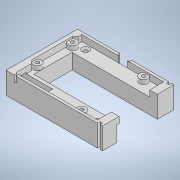
# Autodesk Inventor part: Стойка под электроннику
Saved by Autodesk Inventor 2020 (Build 240168000, 168)
## iProperties
Created: 2021-04-05
Part Number: Стойка под электроннику
Material: Типовые
Document SubType Name: Modeling
Designer: Антон
Density: 1 g/cm^3
Appearance: По умолчанию
Author: Антон
Autodesk Inventor part; units mm, degrees
ref_plane "YZ Plane" through (0, 0, 0) normal (1, 0, 0) x (0, 1, 0)
ref_plane "XZ Plane" through (0, 0, 0) normal (0, 1, 0) x (-1, 0, 0)
ref_plane "XY Plane" through (0, 0, 0) normal (0, 0, 1) x (1, 0, 0)
sketch "Эскиз1" plane through (0, 0, 0) normal (0, 1, 0) x (-1, 0, 0)
  line L0 (0, 0) -> (78, 0)
  line L1 (78, 0) -> (78, -57.8)
  line L2 (78, -57.8) -> (0, -57.8)
  line L3 (0, -57.8) -> (0, 0)
  line L4 (0, -28.9) -> (34.5, -28.9)
  line L5 (69, -13.4) -> (0, -13.4)
  line L6 (0, -13.4) -> (0, -44.4)
  line L7 (0, -44.4) -> (69, -44.4)
  line L8 (69, -44.4) -> (69, -13.4)
  line L9 (69, -13.4) -> (0, -44.4) construction
  line L10 (0, -13.4) -> (69, -44.4) construction
  line L11 (0, -13.4) -> (4, -13.4)
  point P0 (0, -13.4)
  dimension "d0" = 78
  dimension "d1" = 57.8
  dimension "d3" = 31
  dimension "d4" = 69
  constraints: 24 end point, 4 horizontal, 4 parallel, 3 midpoint, 2 perpendicular, 1 point on line
  measures "d0" distance of L1.end L2.end
  measures "d1" distance of L0.end L1.end
  measures "d3" distance of L6.end L5.end
  measures "d4" distance of L6.end L7.end
extrude "Выдавливание1" add sketch "Эскиз1" along normal blind 17.5 contours L0 L1 L2 L3 L7 L8 L5
sketch "Эскиз2" plane through (0, 17.5, 0) normal (0, 1, 0) x (1, 0, 0)
  line L0 (0, 0) -> (0, 2.05)
  line L1 (0, 0) -> (0, 57.8) projected
  line L2 (0, 2.05) -> (-6.2, 2.05)
  line L3 (-6.2, 2.05) -> (-72.4, 2.05)
  line L4 (-72.4, 2.05) -> (-72.4, 55.75)
  line L5 (-72.4, 55.75) -> (-6.2, 55.75)
  line L6 (-6.2, 55.75) -> (-6.2, 2.05)
  line L7 (-72.4, 2.05) -> (-72.4, 17.65)
  line L8 (-72.4, 17.65) -> (-74.9, 17.65)
  line L9 (-74.9, 17.65) -> (-74.9, 50.35)
  line L10 (-74.9, 50.35) -> (-72.4, 50.35)
  line L11 (-72.4, 50.35) -> (-72.4, 17.65)
  line L12 (-78, 57.8) -> (-78, 0) projected
  line L13 (-78, 0) -> (0, 0) projected
  point P0 (0, 11.4)
  point P1 (-72.4, 50.35)
  dimension "d9" = 2.05
  dimension "d10" = 6.2
  dimension "d11" = 66.2
  dimension "d12" = 53.7
  dimension "d13" = 15.6
  dimension "d14" = 2.5
  dimension "d15" = 32.7
  dimension "d16" = 57.8
  dimension "d17" = 78
  constraints: 22 end point, 4 parallel, 3 perpendicular, 2 horizontal, 2 point on line
  measures "d9" distance of L0.start L0.end
  measures "d10" distance of L0.end L2.end
  measures "d11" distance of L4.end L5.end
  measures "d12" distance of L3.end L4.end
  measures "d13" distance of L3.end L7.end
  measures "d14" distance of L9.end L10.end
  measures "d15" distance of L8.end L9.end
  measures "d16" distance of L12.start L12.end
  measures "d17" distance of L12.end L0.start
extrude "Выдавливание2" cut sketch "Эскиз2" against normal blind 5
sketch "Эскиз3" plane through (0, 12.5, 0) normal (0, 1, 0) x (1, 0, 0)
  line L0 (-74.9, 17.65) -> (-74.9, 50.35) projected
  line L1 (-74.9, 50.35) -> (-74.9, 48.15)
  line L2 (-74.9, 48.15) -> (-72.3, 48.15)
  circle A0 centre (-72.3, 48.15) radius 3.5
  line L3 (-74.9, 17.65) -> (-74.9, 19.65)
  line L4 (-74.9, 19.65) -> (-72.3, 19.65)
  circle A1 centre (-72.3, 19.65) radius 3.3
  line L5 (-6.2, 2.05) -> (-72.4, 2.05) projected
  line L6 (-6.2, 55.75) -> (-6.2, 2.05) projected
  line L7 (-6.2, 55.75) -> (-19.8, 55.75)
  line L8 (-72.4, 55.75) -> (-6.2, 55.75) projected
  line L9 (-19.8, 55.75) -> (-19.8, 53.15)
  circle A2 centre (-19.8, 53.15) radius 3.5
  line L10 (-6.2, 2.05) -> (-72.4, 2.05) projected
  line L11 (-6.2, 2.05) -> (-21.3, 2.05)
  line L12 (-21.3, 2.05) -> (-21.3, 4.65)
  circle A3 centre (-21.3, 4.65) radius 3.5
  point P0 (-6.2, 44.4)
  dimension "d26" = 2.2
  dimension "d27" = 2.6
  dimension "d28" = 7
  dimension "d29" = 2
  dimension "d30" = 2.6
  dimension "d31" = 6.6
  dimension "d35" = 13.6
  dimension "d36" = 2.6
  dimension "d37" = 7
  dimension "d38" = 15.1
  dimension "d39" = 2.6
  dimension "d40" = 7
  constraints: 16 end point, 4 centre point, 4 coincident, 4 point on line, 2 horizontal, 2 vertical
  measures "d26" distance of L0.end L1.end
  measures "d27" distance of L1.end L2.end
  measures "d28" diameter of A0
  measures "d29" distance of L0.start L3.end
  measures "d30" distance of L3.end L4.end
  measures "d31" diameter of A1
  measures "d35" distance of L6.start L7.end
  measures "d36" distance of L7.end L9.end
  measures "d37" diameter of A2
  measures "d38" distance of L5.start L11.end
  measures "d39" distance of L11.end L12.end
  measures "d40" diameter of A3
extrude "Выдавливание5" add sketch "Эскиз3" along normal blind 3.5
chamfer "Фаска2" distance 1 angle 45 1 edges at (-72.4, 15, -2.05)
chamfer "Фаска3" distance 2.5 angle 45 2 edges at (-72.4, 16.75, -17.65) (-72.4, 16.75, -50.35)
sketch "Эскиз4" plane through (-71.3, 16, -19.65) normal (0, 1, 0) x (0, 0, -1)
  arc A0 (-17.6, -52.3431) -> (-17.6, -47.6569) centre (-15, -50) ccw projected
  arc A1 (36.1, -49.1569) -> (36.1, -53.8431) centre (33.5, -51.5) ccw projected
  arc A2 (26.1569, 3.6) -> (31.5042, 2.7958) centre (28.5, 1) ccw projected
  arc A3 (-2.6937, 2.9063) -> (2.0322, 3.6) centre (0, 1) ccw projected
  point P0 (-19.65, -71.3)
  point P1 (50.1, -17.6)
  point P2 (51.1, 36.1)
  point P3 (30.0431, 3.6)
  constraints: 3 coincident, 2 other
hole "Отверстие1" at (-21.3, 16, -4.65) at (-19.8, 16, -53.15) at (-72.3, 16, -48.15) at (-72.3, 16, -19.65) direction (0, -1, 0) diameter 3 depth 5
sketch "Эскиз5" plane through (0, 12.5, 0) normal (0, 1, 0) x (1, 0, 0)
  line L0 (-72.4, 55.75) -> (-6.2, 55.75) projected
  line L1 (-6.2, 2.05) -> (-10.2, 2.05)
  line L2 (-10.2, 2.05) -> (-10.2, 6.05)
  line L3 (-6.2, 2.05) -> (-71.4, 2.05) projected
  line L4 (-72.4, 55.75) -> (-65.4, 55.75)
  line L5 (-65.4, 55.75) -> (-65.4, 51.75)
  line L6 (-6.2, 55.75) -> (-6.2, 2.05) projected
  point P0 (-21.2, 2.05)
  point P1 (-6.2, 44.4)
  dimension "d80" = 4
  dimension "d81" = 4
  dimension "d84" = 7
  dimension "d85" = 4
  constraints: 8 end point, 2 perpendicular, 1 horizontal, 1 point on line
  measures "d80" distance of L1.start L1.end
  measures "d81" distance of L1.end L2.end
  measures "d84" distance of L0.start L4.end
  measures "d85" distance of L4.end L5.end
hole "Отверстие2" at (-65.4, 12.5, -51.75) at (-10.2, 12.5, -6.05) direction (0, -1, 0) diameter 3.2 end through all countersink diameter 5.8 countersink angle 90
sketch "Эскиз10" plane through (0, 0, 0) normal (0, -1, 0) x (1, 0, 0)
  line L0 (0, 0) -> (0, -13.4) projected
  line L1 (0, -13.4) -> (-4, -13.4)
  line L2 (-4, -13.4) -> (-4, -11.4)
  line L3 (-4, -11.4) -> (0, -11.4)
  line L4 (0, -11.4) -> (0, -13.4)
  dimension "d109" = 4
  dimension "d110" = 2
  constraints: 8 end point, 2 parallel, 1 horizontal, 1 perpendicular
  measures "d109" distance of L2.end L3.end
  measures "d110" distance of L1.end L2.end
extrude "Выдавливание9" cut sketch "Эскиз10" against normal up to surface (12.5 mm away)
sketch "Эскиз11" plane through (-78, 0, 0) normal (0, 0, 1) x (1, 0, 0)
  line L0 (78, 0) -> (78, 17.5) projected
  line L1 (78, 0) -> (78, 0)
  line L2 (78, 17.5) -> (78, 17.5)
  line L3 (78, 0) -> (76, 0)
  line L4 (78, 17.5) -> (76, 17.5)
  line L5 (76, 0) -> (74, 0)
  line L6 (74, 0) -> (74, 17.5)
  line L7 (74, 17.5) -> (76, 17.5)
  line L8 (76, 17.5) -> (76, 0)
  line L9 (0, 17.5) -> (78, 17.5) projected
  dimension "d113" = 2
  dimension "d115" = 2
  constraints: 16 end point, 3 horizontal, 2 equal length, 2 parallel, 2 point on line, 1 collinear, 1 perpendicular
  measures "d113" distance of L1.end L3.end
  measures "d115" distance between parallel lines of L8 L6
extrude "Выдавливание10" cut sketch "Эскиз11" against normal blind 2 contours L5 L6 L7 L8
ref_plane "РабПлоскость2" through (-78, 0, -28.9) normal (0, 0, 1) x (1, 0, 0)
mirror "Зеркальное отражение1" about plane through (-78, 0, -28.9) normal (0, 0, 1) of "Выдавливание10"
sketch "Эскиз12" plane through (0, 0, 0) normal (0, -1, 0) x (1, 0, 0)
  line L0 (-36, -57.8) -> (-42, -57.8) construction
  line L1 (0, -57.8) -> (-78, -57.8) projected
  line L2 (-36, -55.75) -> (-42, -55.75)
  line L3 (-42, -59.85) -> (-36, -59.85)
  arc A0 (-36, -59.85) -> (-36, -55.75) centre (-36, -57.8) ccw
  arc A1 (-42, -55.75) -> (-42, -59.85) centre (-42, -57.8) ccw
  line L4 (-72.4, -52.85) -> (-74.9, -50.35) projected
  line L5 (-72.4, -52.85) -> (-72.4, -55.75) projected
  line L6 (-72.4, -55.75) -> (-6.2, -55.75) projected
  line L7 (-6.2, -55.75) -> (-6.2, -44.4) projected
  line L8 (-6.2, -44.4) -> (0, -44.4) projected
  line L9 (0, -44.4) -> (0, -57.8) projected
  line L10 (0, -57.8) -> (-2, -57.8) projected
  line L11 (-78, -57.8) -> (-78, 0) projected
  line L12 (-78, 0) -> (-4, 0) projected
  line L13 (0, 0) -> (0, -13.4) projected
  line L14 (0, -13.4) -> (-6.2, -13.4) projected
  line L15 (-6.2, -13.4) -> (-6.2, -2.05) projected
  line L16 (-6.2, -2.05) -> (-71.4, -2.05) projected
  line L17 (-72.4, -3.05) -> (-71.4, -2.05) projected
  line L18 (-72.4, -3.05) -> (-72.4, -15.15) projected
  line L19 (-74.9, -17.65) -> (-72.4, -15.15) projected
  line L20 (-74.9, -17.65) -> (-74.9, -50.35) projected
  line L21 (-36, -55.75) -> (-42, -55.75)
  line L22 (-42, -55.75) -> (-42, -56.75)
  line L23 (-42, -56.75) -> (-36, -56.75)
  line L24 (-36, -56.75) -> (-36, -55.75)
  line L25 (-36, -56.75) -> (-35.5, -56.75)
  line L26 (-35.5, -56.75) -> (-35.5, -55.75)
  line L27 (-35.5, -55.75) -> (-36, -55.75)
  line L28 (-36, -55.75) -> (-36, -56.75)
  line L29 (-42, -56.75) -> (-42.5, -56.75)
  line L30 (-42.5, -56.75) -> (-42.5, -55.75)
  line L31 (-42.5, -55.75) -> (-42, -55.75)
  line L32 (-42, -55.75) -> (-42, -56.75)
  line L33 (-2, -57.8) -> (-2, -55.8) projected
  line L34 (-2, -55.8) -> (-4, -55.8) projected
  line L35 (-4, -55.8) -> (-4, -57.8) projected
  line L36 (-4, -57.8) -> (-78, -57.8) projected
  line L37 (-4, 0) -> (-4, -2) projected
  line L38 (-4, -2) -> (-2, -2) projected
  line L39 (-2, -2) -> (-2, 0) projected
  line L40 (-2, 0) -> (0, 0) projected
  point P0 (-39, -57.8)
  point P1 (-42.5, -55.8119)
  point P2 (-42, -55.75)
  point P3 (-35.5, -55.8119)
  point P4 (-36, -55.75)
  dimension "d118" = 3
  dimension "d125" = 1
  dimension "d126" = 0.5
  constraints: 32 end point, 7 parallel, 4 point on circle, 4 tangent, 3 horizontal, 3 perpendicular, 3 point on line, 2 centre point, 2 collinear, 2 midpoint
  measures "d118" distance of point (-39, -57.8) L0.end
  measures "d125" distance between parallel lines of L2 L23
  measures "d126" distance of L27.end L26.end
extrude "Выдавливание11" cut sketch "Эскиз12" against normal through all contours A0 L3 A1 L1 | L1 A1 L30 L29 L23 L25 L26 A0 | L26 L25 L24 A0 | A0 L6 L26 | L30 L6 A1 | A1 L22 L29 L30 | L24 L23 L22 L2
sketch "Эскиз14" plane through (0, 17.5, 0) normal (0, 1, 0) x (1, 0, 0)
  line L0 (-44.05, 57.8) -> (-78, 57.8) projected
  line L1 (-72.4, 55.75) -> (-42.5, 55.75) projected
  line L2 (-42.5, 55.75) -> (-35.5, 55.75) projected
  line L3 (-39, 55.75) -> (-39, 57)
  line L4 (0, 57.8) -> (-33.95, 57.8) projected
  line L5 (-30.95, 57.8) -> (-28.95, 57.8)
  line L6 (-28.95, 57.8) -> (-28.95, 53.75)
  line L7 (-28.95, 53.75) -> (-30.95, 53.75)
  line L8 (-30.95, 53.75) -> (-30.95, 57.8)
  line L9 (-28.95, 53.75) -> (-49.05, 53.75)
  line L10 (-49.05, 53.75) -> (-49.05, 55.75)
  line L11 (-49.05, 55.75) -> (-28.95, 55.75)
  line L12 (-28.95, 55.75) -> (-28.95, 53.75)
  line L13 (-49.05, 53.75) -> (-47.05, 53.75)
  line L14 (-47.05, 53.75) -> (-47.05, 57.8)
  line L15 (-47.05, 57.8) -> (-49.05, 57.8)
  line L16 (-49.05, 57.8) -> (-49.05, 53.75)
  point P0 (0, 0)
  point P1 (-35.5, 55.8119)
  point P2 (-30.95, 55.75)
  point P3 (-47.05, 55.75)
  dimension "d136" = 2
  dimension "d137" = 2
  dimension "d138" = 3
  constraints: 26 end point, 6 parallel, 3 horizontal, 3 perpendicular, 2 collinear, 2 midpoint, 2 point on line, 1 vertical
  measures "d136" distance between parallel lines of L8 L6
  measures "d137" distance between parallel lines of L11 L9
  measures "d138" distance from line of L4.end L8
ref_plane "РабПлоскость4" through (0, 8.75, 0) normal (0, 1, 0) x (1, 0, 0)
extrude "Выдавливание12" cut sketch "Эскиз14" against normal mid plane 5 from surface at -8.75
chamfer "Фаска5" distance 1 angle 45 4 edges at (-28.95, 8.75, -53.75) (-30.95, 8.75, -55.75) (-47.05, 8.75, -55.75) (-49.05, 8.75, -53.75)
sketch "Эскиз21" plane through (0, 0, 0) normal (0, -1, 0) x (1, 0, 0)
  line L0 (-76, -2.7) -> (-51, -2.7)
  line L1 (-51, -2.7) -> (-51, -10.7)
  line L2 (-51, -10.7) -> (-76, -10.7)
  line L3 (-76, -10.7) -> (-76, -2.7)
  line L4 (-78, 0) -> (-4, 0) projected
  line L5 (-78, -57.8) -> (-78, 0) projected
  point P0 (0, 0)
  dimension "d167" = 8
  dimension "d168" = 25
  dimension "d169" = 2.7
  dimension "d170" = 2
  constraints: 8 end point, 2 parallel, 1 horizontal, 1 perpendicular
  measures "d167" distance of L0.end L1.end
  measures "d168" distance of L1.end L2.end
  measures "d169" distance between parallel lines of L4 L0
  measures "d170" distance between parallel lines of L5 L3
extrude "Выдавливание17" cut sketch "Эскиз21" against normal blind 13.5
sketch "Эскиз22" plane through (-78, 0, -57.8) normal (-1, 0, 0) x (0, 0, 1)
  line L0 (47.1, 0) -> (55.1, 0) projected
  line L1 (47.1, 0) -> (47.1, 13.5) projected
  line L2 (47.1, 13.5) -> (55.1, 13.5) projected
  line L3 (55.1, 0) -> (55.1, 13.5) projected
  line L4 (47.1, 0) -> (47.1, 13.5) projected
  line L5 (47.1, 6.75) -> (55.1, 6.75)
  point P0 (57.8, 0)
  point P1 (51.1, 6.75)
  constraints: 3 midpoint, 2 end point
hole "Отверстие4" at (-78, 6.75, -6.7) direction (1, 0, 0) diameter 6.5 depth 2
sketch "Эскиз25" plane through (0, 17.5, 0) normal (0, 1, 0) x (1, 0, 0)
  line L0 (-72.05, 2.7) -> (-71.4, 2.05) projected
  line L1 (-78, 0) -> (-4, 0) projected
  line L2 (-71.4, 2.05) -> (-69.9, 2.05)
  line L3 (-69.9, 2.05) -> (-69.9, 0)
  line L4 (-69.9, 0) -> (-71.4, 0)
  line L5 (-71.4, 0) -> (-71.4, 2.05)
  point P0 (0, 0)
  dimension "d184" = 1.5
  constraints: 8 end point, 2 parallel, 1 horizontal, 1 perpendicular, 1 point on line
  measures "d184" distance between parallel lines of L3 L5
extrude "Выдавливание19" cut sketch "Эскиз25" against normal up to surface (5 mm away)
sketch "Эскиз26" plane through (0, 0, 0) normal (0, -1, 0) x (1, 0, 0)
  line L0 (-78, -43.9) -> (-75.95, -43.9)
  line L1 (-75.95, -43.9) -> (-75.95, -13.9)
  line L2 (-75.95, -13.9) -> (-78, -13.9)
  line L3 (-78, -13.9) -> (-78, -43.9)
  line L4 (-78, -57.8) -> (-78, 0) projected
  line L5 (-75.95, -43.9) -> (-77, -43.9)
  line L6 (-77, -43.9) -> (-77, -44.95)
  line L7 (-77, -44.95) -> (-75.95, -44.95)
  line L8 (-75.95, -44.95) -> (-75.95, -43.9)
  line L9 (-75.95, -13.9) -> (-77, -13.9)
  line L10 (-77, -13.9) -> (-77, -12.85)
  line L11 (-77, -12.85) -> (-75.95, -12.85)
  line L12 (-75.95, -12.85) -> (-75.95, -13.9)
  point P0 (0, 0)
  point P1 (-78, -28.9)
  point P2 (-77, -13.9)
  dimension "d187" = 2.05
  dimension "d188" = 30
  dimension "d189" = 1.05
  dimension "d190" = 1.05
  dimension "d191" = 1.05
  dimension "d192" = 1.05
  constraints: 24 end point, 6 parallel, 3 horizontal, 3 perpendicular, 2 midpoint
  measures "d187" distance of L2.end L1.end
  measures "d188" distance of L1.end L0.end
  measures "d189" distance of L7.end L6.end
  measures "d190" distance of L6.end L5.end
  measures "d191" distance of L10.end L11.end
  measures "d192" distance of L9.end L10.end
extrude "Выдавливание20" cut sketch "Эскиз26" against normal blind 15
equation "\"d9\" = -0.5 * d12 + 0.5 * d16"
